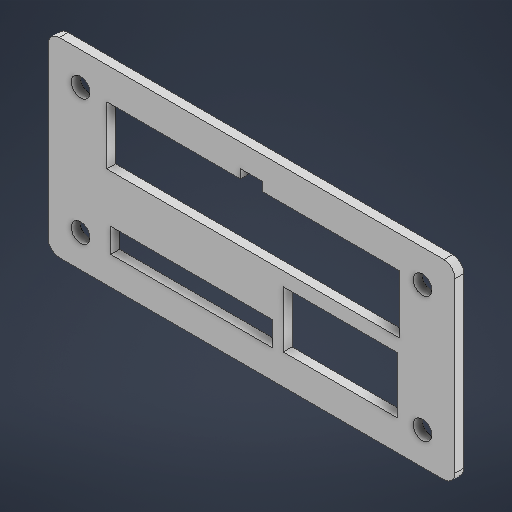
# Autodesk Inventor part: power_sync_module_case_02
Saved by Autodesk Inventor 2026 (Build 300175000, 175)
## iProperties
Created: 2026-03-10
Part Number: power_sync_module_case_02
Material: Generic
Document SubType Name: Modeling
Designer: numai
Density: 1 g/cm^3
Appearance: Default
Author: numai
Autodesk Inventor part; units mm, degrees
ref_plane "YZ Plane" through (0, 0, 0) normal (1, 0, 0) x (0, 1, 0)
ref_plane "XZ Plane" through (0, 0, 0) normal (0, 1, 0) x (-1, 0, 0)
ref_plane "XY Plane" through (0, 0, 0) normal (0, 0, 1) x (1, 0, 0)
sketch "スケッチ1" plane through (0, 0, 0) normal (0, 0, 1) x (1, 0, 0)
  line L0 (-34.52, 15.04) -> (34.52, 15.04) construction
  line L1 (34.52, 15.04) -> (34.52, -15.04) construction
  line L2 (34.52, -15.04) -> (-34.52, -15.04) construction
  line L3 (-34.52, -15.04) -> (-34.52, 15.04) construction
  line L4 (-30.85, 11.35) -> (30.85, 11.35) construction
  line L5 (30.85, 11.35) -> (30.85, -11.35) construction
  line L6 (30.85, -11.35) -> (-30.85, -11.35) construction
  line L7 (-30.85, -11.35) -> (-30.85, 11.35) construction
  circle A0 centre (-30.85, 11.35) radius 1.7
  circle A1 centre (-30.85, -11.35) radius 1.7
  circle A2 centre (30.85, -11.35) radius 1.7
  circle A3 centre (30.85, 11.35) radius 1.7
  line L8 (-25.92, 11.24) -> (26.58, 11.24) construction
  line L9 (26.58, 11.24) -> (26.58, 1.14) construction
  line L10 (26.58, 1.14) -> (-25.92, 1.14) construction
  line L11 (-25.92, 1.14) -> (-25.92, 11.24) construction
  line L12 (-25.22, -7.86) -> (3.58, -7.86) construction
  line L13 (3.58, -7.86) -> (3.58, -11.86) construction
  line L14 (3.58, -11.86) -> (-25.22, -11.86) construction
  line L15 (-25.22, -11.86) -> (-25.22, -7.86) construction
  line L16 (5.92, -1.74) -> (26.12, -1.74) construction
  line L17 (26.12, -1.74) -> (26.12, -11.54) construction
  line L18 (26.12, -11.54) -> (5.92, -11.54) construction
  line L19 (5.92, -11.54) -> (5.92, -1.74) construction
  line L20 (26.78, 0.94) -> (26.78, 11.44)
  line L21 (26.78, 11.44) -> (-26.12, 11.44)
  line L22 (-26.12, 11.44) -> (-26.12, 0.94)
  line L23 (-26.12, 0.94) -> (26.78, 0.94)
  line L24 (3.78, -7.66) -> (-25.42, -7.66)
  line L25 (-25.42, -7.66) -> (-25.42, -12.06)
  line L26 (-25.42, -12.06) -> (3.78, -12.06)
  line L27 (3.78, -12.06) -> (3.78, -7.66)
  line L28 (26.32, -1.54) -> (5.72, -1.54)
  line L29 (5.72, -1.54) -> (5.72, -11.74)
  line L30 (5.72, -11.74) -> (26.32, -11.74)
  line L31 (26.32, -11.74) -> (26.32, -1.54)
  line L32 (-36.7, 17.2) -> (36.7, 17.2)
  line L33 (36.7, 17.2) -> (36.7, -17.2)
  line L34 (36.7, -17.2) -> (-36.7, -17.2)
  line L35 (-36.7, -17.2) -> (-36.7, 17.2)
  line L36 (-2, 11.44) -> (-2, 13.04)
  line L37 (-2, 13.04) -> (2, 13.04)
  line L38 (2, 13.04) -> (2, 11.44)
  point P0 (0, 0)
  point P1 (0, 15.04)
  point P2 (-34.52, 0)
  point P3 (0, 11.35)
  point P4 (-30.85, 0)
  point P5 (-25.22, -9.86)
  point P6 (16.02, -11.54)
  point P7 (0, 17.2)
  point P8 (-36.7, 0)
  point P9 (0, 13.04)
  dimension "d0" = 30.08
  dimension "d1" = 69.04
  dimension "d2" = 61.7
  dimension "d3" = 22.7
  dimension "d4" = 3.4
  dimension "d14" = 3.8
  dimension "d15" = 10.1
  dimension "d16" = 52.5
  dimension "d17" = 8.6
  dimension "d18" = 9.3
  dimension "d19" = 4
  dimension "d20" = 28.8
  dimension "d21" = 3.18
  dimension "d22" = 20.2
  dimension "d23" = 9.8
  dimension "d24" = 8.4
  dimension "d25" = 3.5
  dimension "d26" = 0.2
  dimension "d27" = 0.2
  dimension "d28" = 0.2
  dimension "d29" = 73.4
  dimension "d30" = 34.4
  dimension "d35" = 4
  dimension "d36" = 1.6
  dimension "d33" = 6
  constraints: 78 end point, 18 parallel, 11 perpendicular, 9 midpoint, 6 horizontal, 4 centre point, 4 coincident, 4 vertical alignment, 3 equal radius, 3 horizontal alignment, 2 point on line, 1 vertical, 9 other
  measures "d0" distance of L2.end L0.start
  measures "d1" distance of L0.start L0.end
  measures "d2" distance of L4.start L4.end
  measures "d3" distance of L6.end L4.start
  measures "d4" diameter of A0
  measures "d14" distance between parallel lines of L8 L0
  measures "d15" distance of L10.end L8.start
  measures "d16" distance of L8.start L8.end
  measures "d17" distance between parallel lines of L3 L11
  measures "d18" distance from line of point (-25.22, -9.86) L3
  measures "d19" distance of L14.end L12.start
  measures "d20" distance of L12.start L12.end
  measures "d21" distance between parallel lines of L2 L14
  measures "d22" distance of L17.end L18.end
  measures "d23" distance of L18.end L16.start
  measures "d24" distance between parallel lines of L1 L17
  measures "d25" distance from line of L2 point (16.02, -11.54)
  measures "d26" distance between parallel lines of L9 L20
  measures "d27" distance between parallel lines of L12 L24
  measures "d28" distance between parallel lines of L16 L28
  measures "d29" distance of L32.start L32.end
  measures "d30" distance of L34.end L32.start
  measures "d35" distance of L36.end L37.end
  measures "d36" distance of L37.end L38.end
extrude "押し出し4" add sketch "スケッチ1" along normal blind 1.6
fillet "フィレット1" radius 2 4 edges at (-36.7, 17.2, 0.8) (-36.7, -17.2, 0.8) (36.7, -17.2, 0.8) (36.7, 17.2, 0.8)
